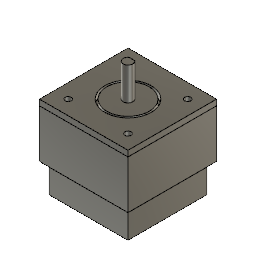
nema-17 v5 (Autodesk Fusion 360 design; units mm, degrees)
Autodesk Fusion 360 part; units mm, degrees
sketch "Sketch1" plane through (0, 0, 0) normal (0, 0, 1) x (1, 0, 0) in component "Nema-17"
  line L0 (20.5, -20.5) -> (-20.5, -20.5)
  line L1 (-20.5, -20.5) -> (-20.5, 20.5)
  line L2 (-20.5, 20.5) -> (20.5, 20.5)
  line L3 (20.5, 20.5) -> (20.5, -20.5)
  line L4 (20.5, -20.5) -> (-20.5, 20.5) construction
  line L5 (-20.5, -20.5) -> (20.5, 20.5) construction
  circle A0 centre (15.5, -15.5) radius 1.6
  circle A1 centre (15.5, 15.5) radius 1.6
  circle A2 centre (-15.5, 15.5) radius 1.6
  circle A3 centre (-15.5, -15.5) radius 1.6
  circle A4 centre (0, 0) radius 11
  circle A5 centre (0, 0) radius 2.5
  circle A6 centre (0, 0) radius 2
  line L6 (0, 2) -> (1.5, 2)
  line L7 (-1.5, 2) -> (1.5, 2)
  dimension "d1" = 41
  dimension "d2" = 41
  dimension "d7" = 3.2
  dimension "d8" = 5
  dimension "d9" = 5
  dimension "d10" = 3.2
  dimension "d11" = 5
  dimension "d12" = 5
  dimension "d13" = 3.2
  dimension "d14" = 5
  dimension "d15" = 5
  dimension "d16" = 3.2
  dimension "d17" = 5
  dimension "d18" = 5
  dimension "d19" = 22
  dimension "d20" = 5
  dimension "d21" = 4
  constraint horizontal L0
  constraint perpendicular L0 L1
  constraint parallel L0 L2
  constraint parallel L1 L3
  constraint coincident L4 A4.centre
  constraint coincident L5 A4.centre
  constraint coincident A4.centre A5.centre
  constraint coincident L4 A0.centre
  constraint concentric A4 A5
  constraint concentric A4 A6
  constraint coincident A6 L6.start
  constraint coincident A5 L6.end
  constraint tangent A6 L6
  constraint horizontal L6
  constraint coincident A5 L7.start
  constraint parallel L6 L7
  measures "d1" distance of L1.end L2.end
  measures "d2" distance of L0.end L1.end
  measures "d7" diameter of A0
  measures "d8" distance of L3 A0.centre
  measures "d9" distance of L0 A0.centre
  measures "d10" diameter of A1
  measures "d11" distance of L2 A1.centre
  measures "d12" distance of L3 A1.centre
  measures "d13" diameter of A2
  measures "d14" distance of L2 A2.centre
  measures "d15" distance of L1 A2.centre
  measures "d16" diameter of A3
  measures "d17" distance of L1 A3.centre
  measures "d18" distance of L0 A3.centre
  measures "d19" diameter of A4
  measures "d20" diameter of A5
  measures "d21" diameter of A6
extrude "Extrude3" add sketch "Sketch1" along normal blind 3 contours A4 makes body 1 in component "Nema-17"
extrude "Extrude2" add sketch "Sketch1" against normal blind 40 separate body contours L0 L1 L2 L3 | A0 | A1 | A2 | A3 | A4 | A6 | A5 L6 L7 | A5 L6 L7 makes body 2 in component "Nema-17"
extrude "Extrude4" cut sketch "Sketch1" against normal blind 10 contours A0 | A1 | A2 | A3 bodies 2 in component "Nema-17"
extrude "Extrude5" add sketch "Sketch1" along normal blind 20 contours A6 | A5 L6 L7 picked at (-1.539, 1.7479) bodies 1 2 in component "Nema-17"
sketch "Sketch1 (2)" plane through (0, 0, 0) normal (0, 0, 1) x (1, 0, 0) in component "joint_cover"
  line L0 (21, -21) -> (-21, -21)
  line L1 (-21, -21) -> (-21, 21)
  line L2 (-21, 21) -> (21, 21)
  line L3 (21, 21) -> (21, -21)
  line L4 (21, -21) -> (-21, 21) construction
  line L5 (-21, -21) -> (21, 21) construction
  line L6 (23, -23) -> (-23, -23)
  line L7 (-23, -23) -> (-23, 23)
  line L8 (-23, 23) -> (23, 23)
  line L9 (23, 23) -> (23, -23)
  line L10 (23, -23) -> (-23, 23) construction
  line L11 (-23, -23) -> (23, 23) construction
  circle A0 centre (0, 0) radius 12
  dimension "d28" = 42
  dimension "d29" = 42
  dimension "d30" = 46
  dimension "d31" = 46
  dimension "d36" = 24
  constraint horizontal L0
  constraint perpendicular L0 L1
  constraint parallel L0 L2
  constraint parallel L1 L3
  constraint coincident L4 A0.centre
  constraint coincident L5 A0.centre
  constraint coincident A0.centre origin
  constraint horizontal L6
  constraint perpendicular L6 L7
  constraint parallel L6 L8
  constraint parallel L7 L9
  constraint coincident L10 A0.centre
  constraint coincident L11 A0.centre
  measures "d28" distance of L1.end L2.end
  measures "d29" distance of L0.end L1.end
  measures "d30" distance of L7.end L8.end
  measures "d31" distance of L6.end L7.end
  measures "d36" diameter of A0
extrude "Extrude2'" add sketch "Sketch1 (2)" along normal blind 3 separate body contours L0 L1 L2 L3 | L6 L7 L8 L9 | A0 makes body 3 in component "joint_cover"
extrude "Extrude1" add sketch "Sketch1 (2)" against normal blind 25 separate body contours L6 L7 L8 L9 makes body 4 in component "joint_cover"
sketch "Sketch2" plane through (0, 0, 3) normal (0, 0, 1) x (-1, 0, 0) in component "joint_cover"
  line L0 (-23, -23) -> (23, -23)
  line L1 (23, -23) -> (23, 23)
  line L2 (23, 23) -> (-23, 23)
  line L3 (-23, 23) -> (-23, -23)
  circle A0 centre (0, 0) radius 12
  circle A1 centre (-15.5, 15.5) radius 1.6
  line L4 (-21, -21) -> (-21, 21)
  line L5 (-21, 21) -> (21, 21)
  circle A2 centre (-15.5, -15.5) radius 1.6
  line L6 (21, -21) -> (-21, -21)
  circle A3 centre (15.5, -15.5) radius 1.6
  line L7 (21, 21) -> (21, -21)
  circle A4 centre (15.5, 15.5) radius 1.6
  dimension "d37" = 24
  dimension "d40" = 3.2
  dimension "d41" = 5.5
  dimension "d42" = 5.5
  dimension "d43" = 3.2
  dimension "d44" = 5.5
  dimension "d45" = 5.5
  dimension "d46" = 3.2
  dimension "d47" = 5.5
  dimension "d48" = 5.5
  dimension "d49" = 3.2
  dimension "d50" = 5.5
  dimension "d51" = 5.5
  constraint coincident A0.centre origin
  measures "d37" diameter of A0
  measures "d40" diameter of A1
  measures "d41" distance of A1.centre L4
  measures "d42" distance of A1.centre L5
  measures "d43" diameter of A2
  measures "d44" distance of L4 A2.centre
  measures "d45" distance of A2.centre L6
  measures "d46" diameter of A3
  measures "d47" distance of A3.centre L7
  measures "d48" distance of L6 A3.centre
  measures "d49" diameter of A4
  measures "d50" distance of L5 A4.centre
  measures "d51" distance of L7 A4.centre
extrude "Extrude3'" cut sketch "Sketch2" against normal up to surface (3 mm away) contours A0 bodies 3 in component "joint_cover"
extrude "Extrude4'" cut sketch "Sketch2" against normal up to surface (3 mm away) contours A1 | A2 | A3 | A4 bodies 3 in component "joint_cover"
component "Nema-17" placed x (1, 0, 0) y (0, 1, 0) z (0, 0, 1) at (0, 0, 0)
component "joint_cover" placed x (1, 0, 0) y (0, 1, 0) z (0, 0, 1) at (0, 0, 0)
